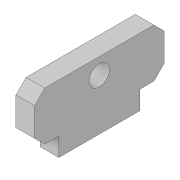
# Autodesk Inventor part: batterywall
Saved by Autodesk Inventor 2017 (Build 210142000, 142)
## iProperties
Created: 2019-06-11
Part Number: batterywall
Material: Generic
Document SubType Name: Modeling
Designer: markg
Density: 1 g/cm^3
Appearance: Default
Author: markg
Autodesk Inventor part; units mm, degrees
ref_plane "YZ Plane" through (0, 0, 0) normal (1, 0, 0) x (0, 1, 0)
ref_plane "XZ Plane" through (0, 0, 0) normal (0, 1, 0) x (-1, 0, 0)
ref_plane "XY Plane" through (0, 0, 0) normal (0, 0, 1) x (1, 0, 0)
sketch "Sketch1" plane through (0, 0, 0) normal (1, 0, 0) x (0, 1, 0)
  line L0 (0, 10.16) -> (7.62, 10.16)
  line L1 (7.62, 10.16) -> (7.62, -10.16)
  line L2 (7.62, -10.16) -> (0, -10.16)
  line L3 (0, -10.16) -> (0, -6.35)
  line L4 (0, -6.35) -> (-2.921, -6.35)
  line L5 (-2.921, -6.35) -> (-2.921, 6.35)
  line L6 (-2.921, 6.35) -> (0, 6.35)
  line L7 (0, 6.35) -> (0, 10.16)
  point P0 (0, 0)
  dimension "d0" = 12.7
  dimension "d1" = 2.921
  dimension "d2" = 20.32
  dimension "d3" = 10.16
  dimension "d4" = 3.81
  dimension "d5" = 7.62
  constraints: 16 end point, 7 perpendicular, 1 horizontal, 1 point on line
  measures "d0" distance of L4.end L5.end
  measures "d1" distance of L3.end L4.end
  measures "d2" distance of L0.end L1.end
  measures "d3" distance from line of point (0, 0) L0
  measures "d4" distance between parallel lines of L0 L6
  measures "d5" distance of L1.end L2.end
extrude "Extrusion1" add sketch "Sketch1" along normal blind 2.921
sketch "Sketch2" plane through (2.921, 0, 0) normal (1, 0, 0) x (0, 0, -1)
  circle A0 centre (0, 5.08) radius 1.5875
  point P0 (0, 0)
  dimension "d8" = 3.175
  dimension "d9" = 5.08
  constraints: 1 centre point
  measures "d8" diameter of A0
  measures "d9" distance of A0.centre point (0, 0)
extrude "Extrusion2" cut sketch "Sketch2" against normal blind 2.921
chamfer "Chamfer1" distance 1.5875 angle 45 4 edges at (1.4605, 7.62, 10.16) (1.4605, 0, 10.16) (1.4605, 7.62, -10.16) (1.4605, 0, -10.16)
body "Solid1"
